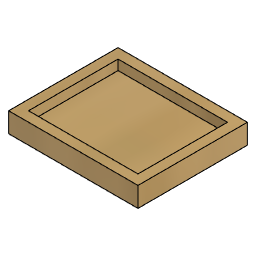
XIAO ESP320S3 Mini (Autodesk Fusion 360 design; units mm, degrees)
Autodesk Fusion 360 part; units mm, degrees
sketch "body" plane through (0, 0, 0) normal (0, 0, 1) x (1, 0, 0)
  line L0 (13, 11) -> (-13, 11)
  line L1 (-13, 11) -> (-13, -11)
  line L2 (-13, -11) -> (13, -11)
  line L3 (13, -11) -> (13, 11)
  line L4 (13, 11) -> (-13, -11) construction
  line L5 (-13, 11) -> (13, -11) construction
  dimension "d2" = 26
  dimension "d3" = 22
  constraint horizontal L0
  constraint perpendicular L0 L1
  constraint parallel L0 L2
  constraint parallel L1 L3
  constraint coincident L4 origin
  constraint coincident L5 origin
  measures "d2" distance of L1.end L2.end
  measures "d3" distance of L0.end L1.end
extrude "Extrude1" add sketch "body" along normal blind 4
sketch "Sketch2" plane through (0, 0, 4) normal (0, 0, 1) x (-1, 0, 0)
  line L0 (-13, 11) -> (-13, -11)
  line L1 (-13, -11) -> (13, -11)
  line L2 (13, -11) -> (13, 11)
  line L3 (13, 11) -> (-13, 11)
  line L4 (13, -11) -> (11, -11)
  line L5 (11, -11) -> (11, -9)
  line L6 (-13, 11) -> (-11, 11)
  line L7 (-11, 11) -> (-11, 9)
  line L8 (11, -9) -> (-11, -9)
  line L9 (-11, -9) -> (-11, 9)
  line L10 (-11, 9) -> (11, 9)
  line L11 (11, 9) -> (11, -9)
  dimension "d6" = 2
  dimension "d7" = 2
  dimension "d8" = 2
  dimension "d9" = 2
  constraint coincident L1.end L2.start
  constraint perpendicular L2 L4
  constraint perpendicular L4 L5
  constraint coincident L0.start L3.end
  constraint perpendicular L0 L6
  constraint perpendicular L6 L7
  constraint horizontal L8
  constraint vertical L9
  constraint horizontal L10
  constraint vertical L11
  measures "d6" distance of L1.end L4.end
  measures "d7" distance of L4.end L5.end
  measures "d8" distance of L0.start L6.end
  measures "d9" distance of L6.end L7.end
extrude "Extrude2" cut sketch "Sketch2" against normal blind 2 contours L8 L9 L10 L11
